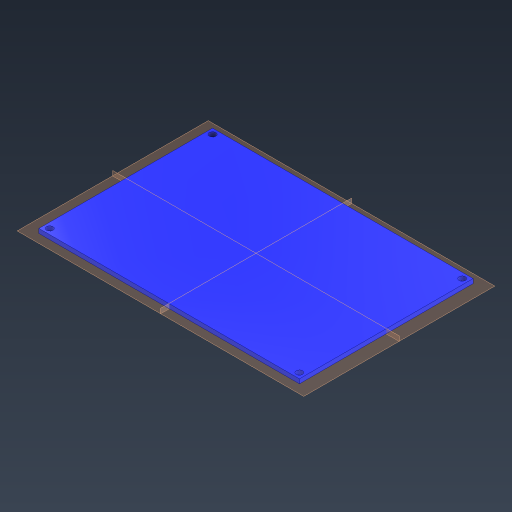
# Autodesk Inventor part: Плата
Saved by Autodesk Inventor 2023.2 (Build 272271030, 271C)
## iProperties
Created: 2025-12-29
Part Number: Плата
Material: Типовые
Document SubType Name: Modeling
Designer: Олег Коноваленко
Density: 1 g/cm^3
Appearance: Синий — малярная краска — глянцевая
Author: Олег Коноваленко
Autodesk Inventor part; units mm, degrees
sketch "Эскиз1" plane through (0, 0, 0) normal (0, 1, 0) x (-1, 0, 0)
  line L0 (60, 40) -> (-60, 40)
  line L1 (-60, 40) -> (-60, -40)
  line L2 (-60, -40) -> (60, -40)
  line L3 (60, -40) -> (60, 40)
  line L4 (60, 40) -> (-60, -40) construction
  line L5 (-60, 40) -> (60, -40) construction
  point P0 (0, 0)
  dimension "d0" = 120
  dimension "d1" = 80
  constraints: 12 end point, 2 midpoint, 2 parallel, 1 horizontal, 1 perpendicular
  measures "d0" distance of L1.end L2.end
  measures "d1" distance of L0.end L1.end
extrude "Выдавливание1" add sketch "Эскиз1" along normal blind 2
sketch "Эскиз2" plane through (0, 2, 0) normal (0, 1, 0) x (1, 0, 0)
  circle A0 centre (-57.5, 37.5) radius 1.5
  line L0 (-60, 40) -> (-60, -40) projected
  line L1 (60, 40) -> (-60, 40) projected
  line L2 (0, 56) -> (0, -56) construction
  line L3 (84, 0) -> (-84, 0) construction
  circle A1 centre (57.5, 37.5) radius 1.5
  circle A2 centre (-57.5, -37.5) radius 1.5
  circle A3 centre (57.5, -37.5) radius 1.5
  dimension "d4" = 3
  dimension "d5" = 2.5
  dimension "d6" = 2.5
  constraints: 4 centre point, 3 symmetric about line, 3 other
  measures "d4" diameter of A0
  measures "d5" distance from line of L0 A0.centre
  measures "d6" distance from line of L1 A0.centre
extrude "Выдавливание2" cut sketch "Эскиз2" against normal up to next
